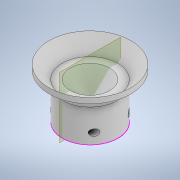
# Autodesk Inventor part: ptfe_catch_135deg
Saved by Autodesk Inventor 2020 (Build 240168000, 168)
## iProperties
Created: 2021-06-26
Part Number: ptfe_catch_135deg
Material: Generic
Document SubType Name: Modeling
Designer: pab2
Density: 1 g/cm^3
Appearance: Default
Author: pab2
Autodesk Inventor part; units mm, degrees
ref_plane "YZ Plane" through (0, 0, 0) normal (1, 0, 0) x (0, 1, 0)
ref_plane "XZ Plane" through (0, 0, 0) normal (0, 1, 0) x (-1, 0, 0)
ref_plane "XY Plane" through (0, 0, 0) normal (0, 0, 1) x (1, 0, 0)
sketch "Sketch1" plane through (0, 0, 0) normal (1, 0, 0) x (0, 1, 0)
  line L0 (0, 0) -> (25.4, 0)
  line L1 (25.4, 0) -> (25.4, -19.05)
  line L2 (25.4, -19.05) -> (0, -19.05)
  line L3 (0, -19.05) -> (0, 0)
  line L4 (0, 0) -> (0, -0.7937)
  line L5 (0, -0.7937) -> (12.7, -0.7937)
  line L6 (12.7, -0.7937) -> (25.4, -13.4937) construction
  line L7 (25.4, -13.4937) -> (25.4, 0)
  line L8 (0, 0) -> (0, -0.7937)
  line L9 (12.7, -0.7937) -> (25.4, -13.4937)
  line L10 (12.7, -0.7937) -> (30.6605, -0.7937) construction
  line L11 (0, -19.05) -> (5.8372, -13.2128)
  line L12 (0, -19.05) -> (8.255, -19.05) construction
  line L13 (25.4, 0) -> (25.4, -18.415)
  line L14 (25.4, -18.415) -> (32.3866, -25.4016)
  line L15 (25.4, -18.415) -> (35.2806, -18.415) construction
  line L16 (32.3866, -25.4016) -> (39.2386, -25.4016)
  line L17 (39.2386, -25.4016) -> (39.2386, 0)
  line L18 (39.2386, 0) -> (25.4, 0)
  line L19 (25.4, -19.05) -> (34.3803, -28.0303)
  line L20 (25.4, -19.05) -> (38.1, -19.05) construction
  line L21 (34.3803, -28.0303) -> (38.1, -28.0303)
  line L22 (0, -19.05) -> (0, -12.7008)
  line L23 (0, -12.7008) -> (25.4, -12.7008)
  line L24 (34.3803, -28.0303) -> (30.6719, -28.0303)
  line L25 (34.3803, -28.0303) -> (38.0887, -28.0303) construction
  line L26 (30.6719, -28.0303) -> (22.3478, -19.05)
  line L27 (25.4, -19.05) -> (22.3478, -19.05)
  point P0 (8.255, 8.255)
  dimension "partH" = 25.4
  dimension "partR" = 19.05
  dimension "tubeID" = 0.7937
  dimension "straightDepth" = 12.7
  dimension "funnelTaperAngle" = 135
  dimension "taperAngle" = 45
  dimension "d15" = 8.255
  dimension "d16" = 45
  dimension "d29" = 18.415
  dimension "d30" = 9.8806
  dimension "d31" = 45
  dimension "d32" = 12.7
  dimension "d33" = 45
  dimension "d34" = 3.7084
  dimension "d35" = 180
  constraints: 56 end point, 9 horizontal, 6 point on line, 5 equal length, 5 perpendicular, 3 parallel, 2 coincident, 1 collinear
  measures "partH" distance of L1.end L2.end
  measures "partR" distance of L0.end L1.end
  measures "tubeID" distance of L0.start L4.end
  measures "straightDepth" distance of L4.end L5.end
  measures "funnelTaperAngle" angle of L5 L6
  measures "taperAngle" angle of L9 L10
  measures "d15" distance of L11.start L11.end
  measures "d16" angle of L12 L11
  measures "d29" distance of L0.end L13.end
  measures "d30" distance of L13.end L14.end
  measures "d31" angle of L14 L15
  measures "d32" distance of L1.end L19.end
  measures "d33" angle of L19 L20
  measures "d34" distance of L19.end L24.end
  measures "d35" angle of L24 L25
revolve "Revolution1" add sketch "Sketch1" angle 360 about axis through (0, 0, 0) along (0, 1, 0) contours L5 L9 L23 L3 | L23 L9 L1 L2 L3 | L2 L19 L24 L26
sketch "Sketch2" plane through (0, 0, 0) normal (0, -1, 0) x (1, 0, 0)
  point P0 (0, 0)
  point P1 (0, 0)
  constraints: 1 coincident
hole "Hole1" at (0, 0, 0) direction (0, 1, 0) diameter 5.3594 depth 9.525 thread size "1/4-28 UNF" class "2B" standard "ANSI Unified Screw Threads"
sketch "Sketch3" plane through (0, 0, 0) normal (0, -1, 0) x (1, 0, 0)
  circle A0 centre (0, 0) radius 0.7937 projected
  line L0 (0, 0) -> (0, -19.05)
  circle A1 centre (0, 0) radius 19.05 projected
  constraints: 2 end point, 1 vertical, 1 vertical alignment, 1 other
ref_plane "Work Plane1" through (0, 0, 0) normal (-1, 0, 0) x (0, 0, -1)
sketch "Sketch4" plane through (0, 0, 0) normal (-1, 0, 0) x (0, 0, -1)
  line L0 (19.05, 0) -> (-19.05, 0) projected
  line L1 (-19.05, 0) -> (-11.8658, -7.1842)
  line L2 (-19.05, 0) -> (-8.89, 0) construction
  line L3 (19.05, 0) -> (11.8658, -7.1842)
  line L4 (19.05, 0) -> (29.21, 0) construction
  point P0 (0, 0)
  dimension "d18" = 10.16
  dimension "d19" = 45
  dimension "d20" = 10.16
  dimension "d21" = 135
  constraints: 8 end point, 2 equal length, 2 horizontal
  measures "d18" distance of L0.end L1.end
  measures "d19" angle of L1 L2
  measures "d20" distance of L0.start L3.end
  measures "d21" angle of L3 L4
hole "Hole2" at (0, 7.1842, 11.8658) at (0, 7.1842, -11.8658) direction (-1, 0, 0) diameter 4.4958 end through all start extended yes clearance for "Flat Head Machine Screw (82)" size "#8" standard "Ansi Unified Screw Threads"
body "Solid1"
